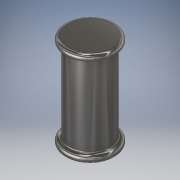
# Autodesk Inventor part: 销钉
Saved by Autodesk Inventor 2019 (Build 230136000, 136)
## iProperties
Created: 2018-12-12
Part Number: 销钉
Material: 钢，高强度，低合金
Document SubType Name: Modeling
Designer: Administrator
Density: 7.85 g/cm^3
Appearance: 钢 - 抛光
Author: Administrator
Autodesk Inventor part; units mm, degrees
ref_plane "YZ Plane" through (0, 0, 0) normal (1, 0, 0) x (0, 1, 0)
ref_plane "XZ Plane" through (0, 0, 0) normal (0, 1, 0) x (-1, 0, 0)
ref_plane "XY Plane" through (0, 0, 0) normal (0, 0, 1) x (1, 0, 0)
sketch "草图1" plane through (0, 0, 0) normal (0, 1, 0) x (-1, 0, 0)
  circle A0 centre (0, 0) radius 30
  dimension "d0" = 60
  constraints: 1 centre point, 1 coincident
  measures "d0" diameter of A0
extrude "拉伸1" add sketch "草图1" along normal blind 120
sketch "草图2" plane through (0, 120, 0) normal (0, 1, 0) x (1, 0, 0)
  circle A0 centre (0, 0) radius 37
  constraints: 1 centre point
extrude "拉伸2" add sketch "草图2" along normal blind 10
sketch "草图3" plane through (0, 0, 0) normal (0, -1, 0) x (1, 0, 0)
  circle A0 centre (0, 0) radius 37
  constraints: 1 centre point
extrude "拉伸3" add sketch "草图3" along normal blind 10
fillet "圆角1" radius 5 4 edges at (-37, 130, 0) (-37, 120, 0) (-37, 0, 0) (-37, -10, 0)
fillet "圆角2" radius 2 2 edges at (30, 120, 0) (30, 0, 0)
